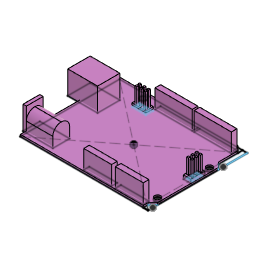
EnclosureForUno (Autodesk Fusion 360 archive; units mm, degrees)
design "ArduinoUno"
Autodesk Fusion 360 part; units mm, degrees
sketch "Sketch1" plane through (0, 0, 0) normal (0, 0, 1) x (1, 0, 0)
  line L0 (34.3, -26.65) -> (-34.3, -26.65)
  line L1 (-34.3, -26.65) -> (-34.3, 26.65)
  line L2 (-34.3, 26.65) -> (29.26, 26.65)
  line L3 (34.3, 26.65) -> (34.3, -26.65)
  line L4 (34.3, -26.65) -> (-34.3, 26.65) construction
  line L5 (-34.3, -26.65) -> (34.3, 26.65) construction
  circle A0 centre (-19, 24.05) radius 1.6
  circle A1 centre (31.8, 8.85) radius 1.6
  circle A2 centre (31.8, -19.05) radius 1.6
  line L6 (31.76, 26.65) -> (34.3, 26.65)
  line L7 (34.3, 26.65) -> (34.3, 13.75)
  line L8 (34.3, 13.75) -> (31.76, 13.75)
  line L9 (31.76, 13.75) -> (31.76, 26.65)
  line L10 (31.76, 13.75) -> (31.76, 13.75)
  line L11 (34.3, 11.21) -> (34.3, -21.56)
  line L12 (31.76, -24.1) -> (31.76, -24.1)
  line L13 (31.76, -24.1) -> (31.76, 13.75) construction
  line L14 (31.76, 13.75) -> (34.3, 11.21)
  line L15 (34.3, -21.56) -> (31.76, -24.1)
  line L16 (31.76, -24.1) -> (34.3, -24.1)
  line L17 (34.3, -24.1) -> (34.3, -26.65)
  line L18 (34.3, -26.65) -> (31.76, -26.65)
  line L19 (31.76, -26.65) -> (31.76, -24.1)
  line L20 (31.76, 26.65) -> (29.22, 26.65)
  line L21 (29.22, 26.65) -> (29.22, 24.11) construction
  line L22 (29.22, 24.11) -> (31.76, 24.11) construction
  line L23 (31.76, 24.11) -> (31.76, 24.15)
  line L24 (29.26, 26.65) -> (31.76, 24.15)
  line L25 (15.26, -22.15) -> (30.26, -22.15)
  line L26 (30.26, -22.15) -> (30.26, -25.15)
  line L27 (30.26, -25.15) -> (15.26, -25.15)
  line L28 (15.26, -25.15) -> (15.26, -22.15)
  line L29 (-1.74, -22.15) -> (13.26, -22.15)
  line L30 (-1.74, -25.15) -> (-1.74, -22.15)
  line L31 (13.26, -25.15) -> (-1.74, -25.15)
  line L32 (13.26, -22.15) -> (13.26, -25.15)
  line L33 (10.26, 25.15) -> (30.26, 25.15)
  line L34 (30.26, 25.15) -> (30.26, 22.15)
  line L35 (30.26, 22.15) -> (10.26, 22.15)
  line L36 (10.26, 22.15) -> (10.26, 25.15)
  line L37 (-10.74, 25.15) -> (9.26, 25.15)
  line L38 (9.26, 25.15) -> (9.26, 22.15)
  line L39 (9.26, 22.15) -> (-10.74, 22.15)
  line L40 (-10.74, 22.15) -> (-10.74, 25.15)
  line L41 (29.3, 4.85) -> (33.3, 4.85)
  line L42 (33.3, 4.85) -> (33.3, -2.65)
  line L43 (33.3, -2.65) -> (29.3, -2.65)
  line L44 (29.3, -2.65) -> (29.3, 4.85)
  line L45 (29.8725, 3.9935) -> (30.8725, 3.9935)
  line L46 (30.8725, 3.9935) -> (30.8725, 2.9935)
  line L47 (30.8725, 2.9935) -> (29.8725, 2.9935)
  line L48 (29.8725, 2.9935) -> (29.8725, 3.9935)
  line L49 (31.7524, 3.0067) -> (31.7524, 4.0067)
  line L50 (32.7524, 3.0067) -> (31.7524, 3.0067)
  line L51 (32.7524, 4.0067) -> (32.7524, 3.0067)
  line L52 (31.7524, 4.0067) -> (32.7524, 4.0067)
  line L53 (29.8988, 0.7719) -> (29.8988, 1.7719)
  line L54 (30.8988, 0.7719) -> (29.8988, 0.7719)
  line L55 (30.8988, 1.7719) -> (30.8988, 0.7719)
  line L56 (29.8988, 1.7719) -> (30.8988, 1.7719)
  line L57 (31.7786, 0.7588) -> (31.7786, 1.7588)
  line L58 (32.7786, 0.7588) -> (31.7786, 0.7588)
  line L59 (32.7786, 1.7588) -> (32.7786, 0.7588)
  line L60 (31.7786, 1.7588) -> (32.7786, 1.7588)
  line L61 (29.8857, -1.5154) -> (29.8857, -0.5154)
  line L62 (30.8857, -1.5154) -> (29.8857, -1.5154)
  line L63 (30.8857, -0.5154) -> (30.8857, -1.5154)
  line L64 (29.8857, -0.5154) -> (30.8857, -0.5154)
  line L65 (31.7786, -1.5154) -> (31.7786, -0.5154)
  line L66 (32.7786, -1.5154) -> (31.7786, -1.5154)
  line L67 (32.7786, -0.5154) -> (32.7786, -1.5154)
  line L68 (31.7786, -0.5154) -> (32.7786, -0.5154)
  line L69 (-40.5, 17.05) -> (-24.5, 17.05)
  line L70 (-24.5, 17.05) -> (-24.5, 5.05)
  line L71 (-24.5, 5.05) -> (-40.5, 5.05)
  line L72 (-40.5, 5.05) -> (-40.5, 17.05)
  line L73 (-36.1, -14.35) -> (-20.1, -14.35)
  line L74 (-20.1, -14.35) -> (-20.1, -23.35)
  line L75 (-20.1, -23.35) -> (-36.1, -23.35)
  line L76 (-36.1, -23.35) -> (-36.1, -14.35)
  line L77 (-18, 21) -> (-10.5, 21)
  line L78 (-10.5, 21) -> (-10.5, 17)
  line L79 (-10.5, 17) -> (-18, 17)
  line L80 (-18, 17) -> (-18, 21)
  line L81 (-17.1612, 20.3412) -> (-16.1612, 20.3412)
  line L82 (-16.1612, 20.3412) -> (-16.1612, 19.3412)
  line L83 (-16.1612, 19.3412) -> (-17.1612, 19.3412)
  line L84 (-17.1612, 19.3412) -> (-17.1612, 20.3412)
  line L85 (-13.7612, 20.3412) -> (-13.7612, 19.3412)
  line L86 (-14.7612, 20.3412) -> (-13.7612, 20.3412)
  line L87 (-14.7612, 19.3412) -> (-14.7612, 20.3412)
  line L88 (-13.7612, 19.3412) -> (-14.7612, 19.3412)
  line L89 (-11.3612, 20.3412) -> (-11.3612, 19.3412)
  line L90 (-12.3612, 20.3412) -> (-11.3612, 20.3412)
  line L91 (-12.3612, 19.3412) -> (-12.3612, 20.3412)
  line L92 (-11.3612, 19.3412) -> (-12.3612, 19.3412)
  line L93 (-17.1612, 18.7531) -> (-16.1612, 18.7531)
  line L94 (-16.1612, 18.7531) -> (-16.1612, 17.7531)
  line L95 (-16.1612, 17.7531) -> (-17.1612, 17.7531)
  line L96 (-17.1612, 17.7531) -> (-17.1612, 18.7531)
  line L97 (-13.7612, 18.7531) -> (-13.7612, 17.7531)
  line L98 (-14.7612, 17.7531) -> (-14.7612, 18.7531)
  line L99 (-14.7612, 18.7531) -> (-13.7612, 18.7531)
  line L100 (-13.7612, 17.7531) -> (-14.7612, 17.7531)
  line L101 (-11.3612, 18.7531) -> (-11.3612, 17.7531)
  line L102 (-12.3612, 17.7531) -> (-12.3612, 18.7531)
  line L103 (-12.3612, 18.7531) -> (-11.3612, 18.7531)
  line L104 (-11.3612, 17.7531) -> (-12.3612, 17.7531)
  point P0 (34.3, 13.75)
  point P1 (34.3, -24.1)
  dimension "d1" = 68.6
  dimension "d2" = 53.3
  dimension "d4" = 3.2
  dimension "d6" = 3.2
  dimension "d7" = 3.2
  dimension "d8" = 15.3
  dimension "d9" = 50.7
  dimension "d10" = 35.5
  dimension "d19" = 12.9
  dimension "d22" = 2.54
  dimension "d23" = 37.85
  dimension "d24" = 2.54
  dimension "d25" = 2.54
  dimension "d26" = 2.54
  dimension "d27" = 2.54
  dimension "d28" = 2.54
  dimension "d29" = 2.54
  dimension "d30" = 2.54
  dimension "d31" = 2.5
  dimension "d32" = 2.5
  dimension "d35" = 15
  dimension "d36" = 3
  dimension "d37" = 1.5
  dimension "d38" = 1.5
  dimension "d39" = 15
  dimension "d40" = 3
  dimension "d41" = 2
  dimension "d42" = 1.5
  dimension "d43" = 20
  dimension "d44" = 3
  dimension "d45" = 20
  dimension "d46" = 3
  dimension "d47" = 1.5
  dimension "d48" = 1.5
  dimension "d49" = 1
  dimension "d50" = 1.5
  dimension "d53" = 4
  dimension "d54" = 7.5
  dimension "d55" = 1
  dimension "d56" = 24
  dimension "d57" = 1
  dimension "d58" = 1
  dimension "d59" = 1
  dimension "d60" = 1
  dimension "d61" = 1
  dimension "d62" = 1
  dimension "d63" = 1
  dimension "d64" = 1
  dimension "d65" = 1
  dimension "d66" = 1
  dimension "d67" = 1
  dimension "d68" = 1
  dimension "d73" = 16
  dimension "d74" = 12
  dimension "d75" = 6.2
  dimension "d76" = 9.6
  dimension "d77" = 16
  dimension "d78" = 9
  dimension "d79" = 3.3
  dimension "d80" = 1.8
  dimension "d87" = 66.1
  dimension "d88" = 7.6
  dimension "d89" = 66.1
  dimension "d90" = 7.5
  dimension "d91" = 4
  dimension "d98" = 1
  dimension "d99" = 1
  dimension "d102" = 4.8
  dimension "d103" = 0
  dimension "d104" = 1
  dimension "d105" = 1
  dimension "d108" = 4.8
  dimension "d109" = 0
  constraint horizontal L0
  constraint perpendicular L0 L1
  constraint parallel L0 L2
  constraint parallel L1 L3
  constraint coincident L4 origin
  constraint coincident L5 origin
  constraint coincident L2 L6.start
  constraint horizontal L6
  constraint vertical L7
  constraint horizontal L8
  constraint vertical L9
  constraint horizontal L10
  constraint vertical L11
  constraint horizontal L12
  constraint vertical L13
  constraint coincident P0 L10
  constraint coincident P0 L11
  constraint coincident L11 P1
  constraint coincident L12 P1
  constraint horizontal L16
  constraint vertical L17
  constraint horizontal L18
  constraint vertical L19
  constraint horizontal L20
  constraint vertical L21
  constraint horizontal L22
  constraint vertical L23
  constraint coincident L6.start L23
  constraint horizontal L25
  constraint vertical L26
  constraint horizontal L27
  constraint vertical L28
  constraint horizontal L29
  constraint vertical L32
  constraint horizontal L31
  constraint vertical L30
  constraint horizontal L33
  constraint vertical L34
  constraint horizontal L35
  constraint vertical L36
  constraint horizontal L37
  constraint vertical L38
  constraint horizontal L39
  constraint vertical L40
  constraint horizontal L41
  constraint vertical L42
  constraint horizontal L43
  constraint vertical L44
  constraint horizontal L45
  constraint vertical L46
  constraint horizontal L47
  constraint vertical L48
  constraint horizontal L52
  constraint vertical L51
  constraint horizontal L50
  constraint vertical L49
  constraint horizontal L56
  constraint vertical L55
  constraint horizontal L54
  constraint vertical L53
  constraint horizontal L60
  constraint vertical L59
  constraint horizontal L58
  constraint vertical L57
  constraint horizontal L64
  constraint vertical L63
  constraint horizontal L62
  constraint vertical L61
  constraint horizontal L68
  constraint vertical L67
  constraint horizontal L66
  constraint vertical L65
  constraint horizontal L69
  constraint vertical L70
  constraint horizontal L71
  constraint vertical L72
  constraint horizontal L73
  constraint vertical L74
  constraint horizontal L75
  constraint vertical L76
  constraint horizontal L77
  constraint vertical L78
  constraint horizontal L79
  constraint vertical L80
  constraint horizontal L81
  constraint vertical L82
  constraint horizontal L83
  constraint vertical L84
  constraint horizontal L93
  constraint vertical L94
  constraint horizontal L95
  constraint vertical L96
  measures "d1" distance of L1.end L3.start
  measures "d2" distance of L0.end L1.end
  measures "d4" diameter of A0
  measures "d6" diameter of A1
  measures "d7" diameter of A2
  measures "d8" distance of L1 A0.centre
  measures "d9" distance of L0 A0.centre
  measures "d10" distance of L0 A1.centre
  measures "d19" distance of L6.start L8.end
  measures "d22" distance of L8.end P0
  measures "d23" distance of L8.end L12.start
  measures "d24" distance of P0 L8.end
  measures "d25" distance of P0 L11.start
  measures "d26" distance of L11.end P1
  measures "d27" distance of L12.start P1
  measures "d28" distance of L12.start P1
  measures "d29" distance of L6.start L20.end
  measures "d30" distance of L6.start L22.end
  measures "d31" distance of L6.start L2.end
  measures "d32" distance of L6.start L23.end
  measures "d35" distance of L25.start L25.end
  measures "d36" distance of L25.start L27.end
  measures "d37" distance of L0 L27
  measures "d38" distance of L19 L26
  measures "d39" distance of L29.start L29.end
  measures "d40" distance of L29.start L30.start
  measures "d41" distance of L28 L32
  measures "d42" distance of L0 L31
  measures "d43" distance of L33.start L33.end
  measures "d44" distance of L33.start L35.end
  measures "d45" distance of L37.start L37.end
  measures "d46" distance of L37.start L39.end
  measures "d47" distance of L2 L33
  measures "d48" distance of L9 L34
  measures "d49" distance of L36 L38
  measures "d50" distance of L2 L37
  measures "d53" distance of L41.start L41.end
  measures "d54" distance of L41.start L43.end
  measures "d55" distance of L3 L42
  measures "d56" distance of L0 L43
  measures "d57" distance of L45.start L45.end
  measures "d58" distance of L45.start L47.end
  measures "d59" distance of L49.end L51.start
  measures "d60" distance of L49.end L49.start
  measures "d61" distance of L53.end L55.start
  measures "d62" distance of L53.end L53.start
  measures "d63" distance of L57.end L59.start
  measures "d64" distance of L57.end L57.start
  measures "d65" distance of L61.end L63.start
  measures "d66" distance of L61.end L61.start
  measures "d67" distance of L65.end L67.start
  measures "d68" distance of L65.end L65.start
  measures "d73" distance of L69.start L69.end
  measures "d74" distance of L69.start L71.end
  measures "d75" distance of L1 L72
  measures "d76" distance of L2 L69
  measures "d77" distance of L73.start L73.end
  measures "d78" distance of L73.start L75.end
  measures "d79" distance of L0 L75
  measures "d80" distance of L1 L76
  measures "d87" distance of L1 A1.centre
  measures "d88" distance of L0 A2.centre
  measures "d89" distance of L1 A2.centre
  measures "d90" distance of L77.start L77.end
  measures "d91" distance of L77.start L79.end
  measures "d98" distance of L81.start L81.end
  measures "d99" distance of L81.start L83.end
  measures "d104" distance of L93.start L93.end
  measures "d105" distance of L93.start L95.end
extrude "Extrude11" add sketch "Sketch1" along normal blind 10.01 contours L81 L82 L83 L84 | L85 L86 L87 L88 | L89 L90 L91 L92 | L93 L94 L95 L96 | L97 L98 L99 L100 | L101 L102 L103 L104 makes body 1 at (-13.7612, 18.4198, 3.3367) makes body 2 at (-11.3612, 18.4198, 3.3367) makes body 3 at (-16.8279, 20.3412, 3.3367) makes body 4 at (-13.7612, 20.0079, 3.3367) makes body 5 at (-11.3612, 20.0079, 3.3367) makes body 6 at (-16.8279, 18.7531, 3.3367)
extrude "Extrude8" add sketch "Sketch1" along normal blind 1 separate body contours L77 L78 L79 L80 | L81 L82 L83 L84 | L85 L86 L87 L88 | L89 L90 L91 L92 | L93 L94 L95 L96 | L97 L98 L99 L100 | L101 L102 L103 L104 makes body 7
extrude "Extrude7" add sketch "Sketch1" along normal blind 10 separate body contours L1 L73 L74 L75 makes body 8
extrude "Extrude6" add sketch "Sketch1" along normal blind 12.5 separate body contours L1 L73 L75 L76 | L1 L69 L71 L72 | L1 L69 L70 L71 makes body 9 at (-29.8333, 5.05, 8.3333) makes body 10 at (-36.1, -20.35, 4.1667)
extrude "Extrude5" add sketch "Sketch1" along normal blind 10.01 separate body contours L45 L46 L47 L48 | L49 L50 L51 L52 | L53 L54 L55 L56 | L57 L58 L59 L60 | L61 L62 L63 L64 | L65 L66 L67 L68 makes body 11 at (30.2322, 1.7719, 3.3367) makes body 12 at (30.2059, 3.9935, 3.3367) makes body 13 at (30.219, -0.5154, 3.3367) makes body 14 at (32.112, 1.7588, 3.3367) makes body 15 at (32.0857, 4.0067, 3.3367) makes body 16 at (32.112, -0.5154, 3.3367)
extrude "Extrude4" add sketch "Sketch1" along normal blind 2 separate body contours L41 L42 L43 L44 makes body 17
extrude "Extrude3" add sketch "Sketch1" along normal blind 10.01 separate body contours L25 L26 L27 L28 | L29 L30 L31 L32 | L33 L34 L35 L36 | L37 L38 L39 L40 makes body 18 at (16.9267, 25.15, 6.6733) makes body 19 at (3.26, -22.15, 3.3367) makes body 20 at (-4.0733, 25.15, 6.6733) makes body 21 at (20.26, -22.15, 3.3367)
extrude "Extrude2" add sketch "Sketch1" along normal blind 1 separate body contours L0 L1 L2 L3 L9 L11 L14 L15 L19 L20 L23 L24 L69 L70 L71 L73 L74 L75 | L1 L73 L74 L75 | L1 L69 L70 L71 | L25 L26 L27 L28 | L29 L30 L31 L32 | L33 L34 L35 L36 | L37 L38 L39 L40 | L41 L42 L43 L44 | L45 L46 L47 L48 | L49 L50 L51 L52 | L53 L54 L55 L56 | L57 L58 L59 L60 | L61 L62 L63 L64 | L65 L66 L67 L68 | L77 L78 L79 L80 | L81 L82 L83 L84 | L85 L86 L87 L88 | L89 L90 L91 L92 | L93 L94 L95 L96 | L97 L98 L99 L100 | L101 L102 L103 L104 makes body 22
sketch "Sketch2" plane through (0, 0, 1) normal (0, 0, 1) x (-1, 0, 0)
  circle A0 centre (-31.8, -8.85) radius 1.6
  circle A1 centre (-31.8, 19.05) radius 1.6
  circle A2 centre (19, -24.05) radius 1.6
  line L0 (-31.76, 26.65) -> (-31.76, 24.1)
  line L1 (-31.76, 24.1) -> (-34.3, 21.56)
  line L2 (-34.3, 21.56) -> (-34.3, -11.21)
  line L3 (-34.3, -11.21) -> (-31.76, -13.75)
  line L4 (-31.76, -13.75) -> (-31.76, -24.15)
  line L5 (-31.76, -24.15) -> (-29.26, -26.65)
  line L6 (-29.26, -26.65) -> (34.3, -26.65)
  line L7 (34.3, -26.65) -> (34.3, 26.65)
  line L8 (34.3, 26.65) -> (-31.76, 26.65)
fillet "Fillet1" radius 4.5 2 edges at (-27.2, -23.35, 10) (-27.2, -14.35, 10) on bodies 8
extrude "Extrude9" add 1 faces at (-15.5, 19.6667, 1) along direction (0, 0, 1) blind 2 on bodies 7 bodies 7 22
extrude "Extrude10" cut 1 faces at (-15.5, 19.6667, 3) along direction (0, 0, -1) blind 1 on bodies 7 bodies 7
equation "d32 = d31"
